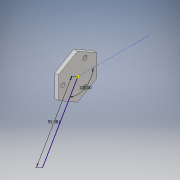
# Autodesk Inventor part: 80_20_Connector
Saved by Autodesk Inventor 2019.4 (Build 234330000, 330)
## iProperties
Created: 2019-07-24
Part Number: 80_20_Connector
Material: Generic
Document SubType Name: Modeling
Designer: Jorian Brusind
Density: 1 g/cm^3
Appearance: Default
Author: Jorian Brusind
Autodesk Inventor part; units mm, degrees
ref_plane "YZ Plane" through (0, 0, 0) normal (1, 0, 0) x (0, 1, 0)
ref_plane "XZ Plane" through (0, 0, 0) normal (0, 1, 0) x (-1, 0, 0)
ref_plane "XY Plane" through (0, 0, 0) normal (0, 0, 1) x (1, 0, 0)
sketch "Sketch5" plane through (0, 0, 0) normal (1, 0, 0) x (0, 1, 0)
  circle A0 centre (0, 0) radius 30
  line L0 (0, 0) -> (30, 0)
  line L1 (30, 0) -> (15, 25.9808)
  line L2 (30, 0) -> (60, 0) construction
  line L3 (15, 25.9808) -> (-15, 25.9808)
  line L4 (-15, 25.9808) -> (-30, 0)
  line L5 (-30, 0) -> (-15, -25.9808)
  line L6 (-15, -25.9808) -> (15, -25.9808)
  line L7 (15, -25.9808) -> (30, 0)
  dimension "d24" = 60
  dimension "d25" = 120
  dimension "d26" = 120
  constraints: 16 end point, 6 point on circle, 2 horizontal, 2 parallel, 1 centre point, 1 coincident, 1 equal length, 1 point on line
  measures "d24" diameter of A0
  measures "d25" angle of L2 L1
  measures "d26" angle of L3 L1
extrude "Extrusion5" add sketch "Sketch5" along normal blind 5 contours L7 L6 L5 L4 L3 L1
sketch "Sketch6" plane through (5, 0, 0) normal (1, 0, 0) x (0, 0, -1)
  line L0 (0, 0) -> (10, 17.3205)
  line L1 (25.9808, 15) -> (0, 30) projected
  line L2 (0, 0) -> (20, 0) construction
  line L3 (0, 0) -> (10, -17.3205)
  line L4 (0, 0) -> (20, 0) construction
  line L5 (0, 0) -> (-20, 0)
  circle A0 centre (10, 17.3205) radius 2.75
  circle A1 centre (-20, 0) radius 2.75
  circle A2 centre (10, -17.3205) radius 2.75
  dimension "d29" = 20
  dimension "d30" = 60
  dimension "d31" = 20
  dimension "d32" = 60
  dimension "d33" = 20
  dimension "d34" = 5.5
  dimension "d35" = 5.5
  dimension "d36" = 5.5
  constraints: 10 end point, 3 centre point, 3 coincident, 2 equal length, 2 horizontal, 1 perpendicular, 1 point on line
  measures "d29" distance of L0.start L0.end
  measures "d30" angle of L2 L0
  measures "d31" distance of L0.start L3.end
  measures "d32" angle of L3 L4
  measures "d33" distance of L0.start L5.end
  measures "d34" diameter of A0
  measures "d35" diameter of A1
  measures "d36" diameter of A2
extrude "Extrusion6" cut sketch "Sketch6" against normal blind 5
sketch "Sketch7" plane through (5, 0, 0) normal (1, 0, 0) x (0, 0, -1)
  circle A0 centre (0, 0) radius 1.5
  dimension "d39" = 3
  constraints: 1 centre point, 1 coincident
  measures "d39" diameter of A0
extrude "Extrusion7" cut sketch "Sketch7" against normal blind 5
sketch "Sketch8" plane through (5, 0, 0) normal (1, 0, 0) x (0, 0, -1)
  circle A0 centre (0, 0) radius 1.5 projected
  line L0 (0, 0) -> (-47.9905, -83.122)
  line L1 (0, 0) -> (95.981, 0) construction
  dimension "d42" = 95.981
  dimension "d43" = 120
  constraints: 4 end point, 1 equal length, 1 horizontal
  measures "d42" distance of L0.start L0.end
  measures "d43" angle of L0 L1
body "Solid2"
